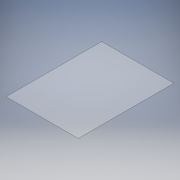
# Autodesk Inventor part: coffeeWindowFrontLeft
Saved by Autodesk Inventor 2019 (Build 230136000, 136)
## iProperties
Created: 2018-09-20
Part Number: coffeeWindowFrontLeft
Material: Glass
Document SubType Name: Modeling
Designer: wade
Density: 2.18 g/cm^3
Appearance: Clear - Light
Author: wade
Autodesk Inventor part; units mm, degrees
ref_plane "YZ Plane" through (0, 0, 0) normal (1, 0, 0) x (0, 1, 0)
ref_plane "XZ Plane" through (0, 0, 0) normal (0, 1, 0) x (-1, 0, 0)
ref_plane "XY Plane" through (0, 0, 0) normal (0, 0, 1) x (1, 0, 0)
sketch "Sketch1" plane through (0, 0, 0) normal (0, 1, 0) x (-1, 0, 0)
  line L0 (0, 0) -> (3100, 0)
  line L1 (3100, 0) -> (3100, -4100)
  line L2 (3100, -4100) -> (0, -4100)
  line L3 (0, -4100) -> (0, 0)
  dimension "d0" = 4100
  dimension "d1" = 3100
  constraints: 8 end point, 2 parallel, 1 horizontal, 1 perpendicular
  measures "d0" distance of L0.end L1.end
  measures "d1" distance of L1.end L2.end
extrude "Extrusion1" add sketch "Sketch1" along normal blind 10
body "Solid1"
